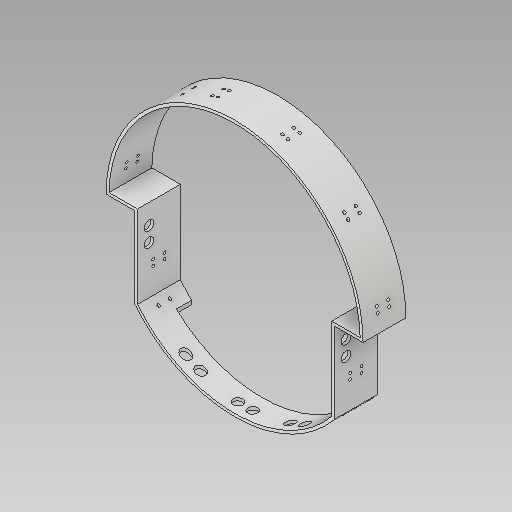
# Autodesk Inventor part: CW000
Saved by Autodesk Inventor 2017 (Build 210142000, 142)
## iProperties
Created: 2017-05-15
Part Number: CW000
Material: ABS Plastic
Document SubType Name: Modeling
Designer: zallen
Density: 1.06 g/cm^3
Appearance: CR White
Author: zallen
Autodesk Inventor part; units mm, degrees
sketch "Sketch1" plane through (0, 0, 0) normal (0, 0, 1) x (1, 0, 0)
  line L0 (-225, 0) -> (-175, 0) construction
  line L1 (-175, 0) -> (-175, -141.4214) construction
  line L2 (225, 0) -> (175, 0) construction
  line L3 (175, 0) -> (175, -141.4214) construction
  arc A0 (225, 0) -> (-225, 0) centre (0, 0) ccw
  arc A1 (-175, -141.4214) -> (175, -141.4214) centre (0, 0) ccw
  line L4 (-225, 0) -> (-175, 0)
  line L5 (-175, -141.4214) -> (-175, 0)
  line L6 (225, 0) -> (175, 0)
  line L7 (175, -141.4214) -> (175, 0)
  arc A2 (219.9432, 5) -> (-219.9432, 5) centre (0, 0) ccw
  line L8 (219.9432, 5) -> (170, 5)
  line L9 (170, 5) -> (170, -139.6424)
  arc A3 (-170, -139.6424) -> (170, -139.6424) centre (0, 0) ccw
  line L10 (-170, -139.6424) -> (-170, 5)
  line L11 (-170, 5) -> (-219.9432, 5)
  dimension "d1" = 50
  dimension "d2" = 50
  dimension "d3" = 5
  constraints: 24 end point, 8 point on circle, 4 centre point, 4 perpendicular, 3 collinear, 2 horizontal, 5 other
  measures "d1" distance of L0.start L0.end
  measures "d2" distance of L2.start L2.end
  measures "d3" radial gap between concentric circles of A0 A2
extrude "Extrusion1" add sketch "Sketch1" along normal blind 75
sketch "Sketch3" plane through (-175, -141.4214, 0) normal (-1, 0, 0) x (0, 0, 1)
  circle A0 centre (47.5, 46.6338) radius 2.5 projected
  circle A1 centre (47.5, 56.6338) radius 2.5 projected
  circle A2 centre (27.5, 56.6338) radius 2.5 projected
  circle A3 centre (27.5, 46.6338) radius 2.5 projected
  circle A4 centre (47.5, 46.6338) radius 2.5
  circle A5 centre (47.5, 56.6338) radius 2.5
  circle A6 centre (27.5, 56.6338) radius 2.5
  circle A7 centre (27.5, 46.6338) radius 2.5
  point P0 (0, 141.4214)
  constraints: 4 centre point, 4 coincident, 4 concentric
extrude "Extrusion2" cut sketch "Sketch3" against normal through all
ref_plane "Work Plane1" through (271.8246, -312.2554, -25.989) normal (0.9877626, 0.1559646, 0) x (-0.0539452, 0.3416485, -0.9382783)
sketch "Sketch4" plane through (271.8246, -312.2554, -25.989) normal (0.9877626, 0.1559646, 0) x (-0.0539452, 0.3416485, -0.9382783)
  circle A0 centre (50.5118, 349.4932) radius 2.5 projected
  circle A1 centre (53.9706, 358.876) radius 2.5 projected
  circle A2 centre (69.2773, 342.5756) radius 2.5 projected
  circle A3 centre (72.7362, 351.9583) radius 2.5 projected
  circle A4 centre (50.5118, 349.4932) radius 2.5
  circle A5 centre (53.9706, 358.876) radius 2.5
  circle A6 centre (69.2773, 342.5756) radius 2.5
  circle A7 centre (72.7362, 351.9583) radius 2.5
  point P0 (96.9603, 338.1646)
  constraints: 4 centre point, 4 coincident, 4 concentric
extrude "Extrusion3" cut sketch "Sketch4" along normal through all
ref_plane "Work Plane2" through (-1525.7616, 1972.576, 1129.6073) normal (0.733942, 0.6792121, 0) x (-0.5490499, 0.5932915, -0.5886844)
sketch "Sketch5" plane through (-1525.7616, 1972.576, 1129.6073) normal (0.733942, 0.6792121, 0) x (-0.5490499, 0.5932915, -0.5886844)
  circle A0 centre (-1378.6077, -2342.6014) radius 2.5 projected
  circle A1 centre (-1370.5241, -2336.7146) radius 2.5 projected
  circle A2 centre (-1366.834, -2358.7687) radius 2.5 projected
  circle A3 centre (-1358.7504, -2352.8819) radius 2.5 projected
  circle A4 centre (-1378.6077, -2342.6014) radius 2.5
  circle A5 centre (-1370.5241, -2336.7146) radius 2.5
  circle A6 centre (-1366.834, -2358.7687) radius 2.5
  circle A7 centre (-1358.7504, -2352.8819) radius 2.5
  point P0 (-1343.0497, -2375.4673)
  constraints: 4 centre point, 4 coincident, 4 concentric
extrude "Extrusion4" cut sketch "Sketch5" along normal through all
ref_plane "Work Plane3" through (1434.1865, -177.8751, -459.6919) normal (0.2726306, 0.9621188, 0) x (-0.9437667, 0.2674302, 0.1943847)
sketch "Sketch6" plane through (1434.1865, -177.8751, -459.6919) normal (0.2726306, 0.9621188, 0) x (-0.9437667, 0.2674302, 0.1943847)
  circle A0 centre (1494.7924, 220.8397) radius 2.5 projected
  circle A1 centre (1504.6016, 218.8958) radius 2.5 projected
  circle A2 centre (1490.9047, 201.2212) radius 2.5 projected
  line L0 (1490.4637, 173.2738) -> (1505.0426, 246.8432) projected
  circle A3 centre (1500.714, 199.2773) radius 2.5 projected
  line L1 (1512.1992, 168.9666) -> (1526.7781, 242.536) projected
  circle A4 centre (1494.7924, 220.8397) radius 2.5
  circle A5 centre (1504.6016, 218.8958) radius 2.5
  circle A6 centre (1500.714, 199.2773) radius 2.5
  circle A7 centre (1490.9047, 201.2212) radius 2.5
  constraints: 4 centre point, 4 coincident, 4 concentric
extrude "Extrusion5" cut sketch "Sketch6" along normal through all
ref_plane "Work Plane4" through (-4192.191, -959.3964, 357.9649) normal (-0.2726306, 0.9621188, 0) x (0.3789755, 0.1073883, -0.9191547)
sketch "Sketch7" plane through (-4192.191, -959.3964, 357.9649) normal (-0.2726306, 0.9621188, 0) x (0.3789755, 0.1073883, -0.9191547)
  circle A0 centre (1975.1614, -3820.8333) radius 2.5 projected
  circle A1 centre (1979.1004, -3830.0249) radius 2.5 projected
  circle A2 centre (1997.4835, -3822.1469) radius 2.5 projected
  circle A3 centre (1993.5445, -3812.9554) radius 2.5 projected
  circle A4 centre (1975.1614, -3820.8333) radius 2.5
  circle A5 centre (1993.5445, -3812.9554) radius 2.5
  circle A6 centre (1997.4835, -3822.1469) radius 2.5
  circle A7 centre (1979.1004, -3830.0249) radius 2.5
  point P0 (2020.7908, -3806.719)
  constraints: 4 centre point, 4 coincident, 4 concentric
extrude "Extrusion6" cut sketch "Sketch7" along normal through all
ref_plane "Work Plane5" through (1559.4764, -1635.2314, 273.0978) normal (0.7236707, 0.6901454, 0) x (0.3635204, -0.3811792, -0.8500325)
sketch "Sketch8" plane through (1559.4764, -1635.2314, 273.0978) normal (0.7236707, 0.6901454, 0) x (0.3635204, -0.3811792, -0.8500325)
  circle A0 centre (-1115.5243, 2228.5218) radius 2.5
  circle A1 centre (-1098.5236, 2239.0564) radius 2.5
  circle A2 centre (-1093.2563, 2230.5561) radius 2.5
  circle A3 centre (-1110.257, 2220.0215) radius 2.5
  ellipse E0 centre (-1114.5854, 2227.0066) end of major axis (-1112.4603, 2228.3234) minor radius 0.1469 projected
  ellipse E1 centre (-1097.5847, 2237.5412) end of major axis (-1095.4596, 2238.858) minor radius 0.1469 projected
  ellipse E2 centre (-1114.2758, 2226.5069) end of major axis (-1116.4008, 2225.1901) minor radius 0.1469 projected
  ellipse E3 centre (-1097.2751, 2237.0415) end of major axis (-1099.4002, 2235.7247) minor radius 0.1469 projected
  point P0 (-958.0758, 2064.6117)
  constraints: 4 centre point, 8 other
extrude "Extrusion7" cut sketch "Sketch8" along normal through all contours E0 A0 | A0 E0 | E0 A0 | E2 A0 | A0 E2 | E1 A1 | A1 E1 | E1 A1 | E3 A1 | A1 E3 picked at (-1114.0777, 2227.3775) picked at (-1116.4263, 2225.8983) picked at (-1112.9086, 2228.0801) picked at (-1097.077, 2237.9121) picked at (-1099.4256, 2236.4329) picked at (-1095.9079, 2238.6147)
ref_plane "Work Plane6" through (-504.1513, -1801.6809, 555.963) normal (-0.9880034, 0.154432, 0) x (0.1211937, 0.7753562, 0.6197861)
sketch "Sketch9" plane through (-504.1513, -1801.6809, 555.963) normal (-0.9880034, 0.154432, 0) x (0.1211937, 0.7753562, 0.6197861)
  circle A0 centre (1146.8301, 1553.6413) radius 2.5 projected
  circle A1 centre (1138.9824, 1547.4434) radius 2.5 projected
  circle A2 centre (1134.4344, 1569.3367) radius 2.5 projected
  circle A3 centre (1126.5867, 1563.1388) radius 2.5 projected
  circle A4 centre (1138.9824, 1547.4434) radius 2.5
  circle A5 centre (1126.5867, 1563.1388) radius 2.5
  circle A6 centre (1134.4344, 1569.3367) radius 2.5
  circle A7 centre (1146.8301, 1553.6413) radius 2.5
  point P0 (1113.4664, 1587.819)
  constraints: 4 centre point, 4 coincident, 4 concentric
extrude "Extrusion8" cut sketch "Sketch9" along normal through all
ref_plane "Work Plane7" through (-593.0618, 311.3539, -544.5578) normal (-0.7298307, -0.683628, 0) x (-0.6824701, 0.7285946, 0.0581765)
sketch "Sketch10" plane through (-593.0618, 311.3539, -544.5578) normal (-0.7298307, -0.683628, 0) x (-0.6824701, 0.7285946, 0.0581765)
  circle A0 centre (-597.0986, -627.8583) radius 2.5 projected
  circle A1 centre (-598.2622, -607.8921) radius 2.5 projected
  circle A2 centre (-597.0986, -627.8583) radius 2.5
  circle A3 centre (-598.2622, -607.8921) radius 2.5
  point P0 (-599.9173, -580.4419)
  constraints: 2 centre point, 2 coincident, 2 concentric
extrude "Extrusion9" cut sketch "Sketch10" along normal through all
ref_plane "Work Plane8" through (437.4356, 145.0915, 442.8518) normal (0.7298307, -0.683628, 0) x (0.006167, 0.0065837, -0.9999593)
sketch "Sketch11" plane through (437.4356, 145.0915, 442.8518) normal (0.7298307, -0.683628, 0) x (0.006167, 0.0065837, -0.9999593)
  circle A0 centre (391.6825, -408.5163) radius 2.5 projected
  circle A1 centre (411.6817, -408.6967) radius 2.5 projected
  circle A2 centre (391.6825, -408.5163) radius 2.5
  circle A3 centre (411.6817, -408.6967) radius 2.5
  point P0 (439.1809, -408.9139)
  constraints: 2 centre point, 2 coincident, 2 concentric
extrude "Extrusion10" cut sketch "Sketch11" along normal through all
ref_plane "Work Plane9" through (-170, -139.6424, 0) normal (0.0051563, 0.9999867, 0) x (0, 0, 1)
sketch "Sketch12" plane through (-170, -139.6424, 0) normal (0.0051563, 0.9999867, 0) x (0, 0, 1)
  line L0 (0, 0) -> (0, 339.9955) projected
  line L1 (0, 20) -> (27, 20)
  line L2 (27, 20) -> (27, 320)
  line L3 (27, 320) -> (0, 320)
  line L4 (0, 320) -> (0, 20)
  point P0 (0, 169.2777)
  dimension "d24" = 27
  dimension "d25" = 20
  dimension "d26" = 300
  constraints: 8 end point, 2 parallel, 1 horizontal, 1 perpendicular, 1 point on line
  measures "d24" distance of L3.end L2.end
  measures "d25" distance from line of L0.start L1
  measures "d26" distance of L1.end L2.end
extrude "Extrusion11" cut sketch "Sketch12" against normal through all
sketch "Sketch13" plane through (175, -141.4214, 0) normal (1, 0, 0) x (0, 0, -1)
  circle A0 centre (-55, 85.4214) radius 8.5
  circle A1 centre (-55, 111.4214) radius 8.5
  line L0 (0, 141.4214) -> (0, 0) projected
  line L1 (0, 141.4214) -> (-75, 141.4214) projected
  dimension "d29" = 17
  dimension "d30" = 17
  dimension "d31" = 26
  dimension "d32" = 55
  dimension "d35" = 30
  constraints: 2 centre point, 1 vertical alignment
  measures "d29" diameter of A0
  measures "d30" diameter of A1
  measures "d31" distance of A1.centre A0.centre
  measures "d32" distance from line of L0 A0.centre
  measures "d35" distance from line of L1 A1.centre
extrude "Extrusion12" cut sketch "Sketch13" against normal through all
sketch "Sketch14" plane through (-170, -139.6424, 0) normal (0.0051563, 0.9999867, 0) x (0, 0, 1)
  circle A0 centre (55, 64.7777) radius 8.5
  circle A1 centre (55, 90.7777) radius 8.5
  circle A2 centre (55, 247.7777) radius 8.5
  circle A3 centre (55, 273.7777) radius 8.5
  circle A4 centre (55, 156.2777) radius 8.5
  circle A5 centre (55, 182.2777) radius 8.5
  point P0 (0, 169.2777)
  dimension "d36" = 17
  dimension "d37" = 17
  dimension "d38" = 26
  dimension "d39" = 17
  dimension "d40" = 17
  dimension "d41" = 26
  dimension "d45" = 17
  dimension "d46" = 17
  dimension "d47" = 26
  dimension "d49" = 13
  dimension "d50" = 65.5
  dimension "d51" = 65.5
  dimension "d52" = 55
  constraints: 6 centre point, 5 vertical alignment
  measures "d36" diameter of A0
  measures "d37" diameter of A1
  measures "d38" distance of A1.centre A0.centre
  measures "d39" diameter of A2
  measures "d40" diameter of A3
  measures "d41" distance of A3.centre A2.centre
  measures "d45" diameter of A4
  measures "d46" diameter of A5
  measures "d47" distance of A5.centre A4.centre
  measures "d49" vertical distance of point (0, 169.278) A4.centre
  measures "d50" distance of A4.centre A1.centre
  measures "d51" distance of A2.centre A5.centre
  measures "d52" horizontal distance of point (0, 169.278) A2.centre
extrude "Extrusion13" cut sketch "Sketch14" against normal through all
body "Solid1"
